Autodesk Fusion 360 part; units mm, degrees
note: some values were not read from the file. Chosen so that the rebuilt part matches the saved one: which bodies a step acts on; that a step has no effect; a side. Set by a fixed rule: which sketch regions a step uses.
(part 2 of 2)
sketch "Schizzo1 (12)" plane through (-2.8, 0, 0) normal (1, 0, 0) x (0, 1, 0) in component "spring"
  line L0 (37.6, 14) -> (48, 14) construction
  line L1 (48, 14) -> (48, 3.6) construction
  line L2 (48, 3.6) -> (37.6, 3.6)
  line L3 (37.6, 3.6) -> (37.6, 14) construction
  line L4 (39.4, 4.4) -> (46.2, 4.4)
  arc A0 (46.2, 4.4) -> (46.2, 6) centre (46.2, 5.2) ccw
  line L5 (46.2, 6) -> (39.4, 6)
  arc A1 (39.4, 6) -> (39.4, 4.4) centre (39.4, 5.2) ccw
  line L6 (39.4, 5.2) -> (46.2, 5.2) construction
  line L7 (46.2, 6.8) -> (39.4, 6.8)
  arc A2 (39.4, 6.8) -> (39.4, 3.6) centre (39.4, 5.2) ccw
  line L8 (39.4, 3.6) -> (46.2, 3.6)
  arc A3 (46.2, 3.6) -> (46.2, 6.8) centre (46.2, 5.2) ccw
  line L9 (42.8, 14) -> (42.8, 3.6) construction
  arc A4 (39.4, 9.2) -> (39.4, 6) centre (39.4, 7.6) ccw
  line L10 (39.4, 6) -> (46.2, 6)
  arc A5 (46.2, 6) -> (46.2, 9.2) centre (46.2, 7.6) ccw
  line L11 (46.2, 9.2) -> (39.4, 9.2)
  arc A6 (46.2, 6.8) -> (46.2, 8.4) centre (46.2, 7.6) ccw
  line L12 (46.2, 8.4) -> (39.4, 8.4)
  arc A7 (39.4, 8.4) -> (39.4, 6.8) centre (39.4, 7.6) ccw
  line L13 (39.4, 6.8) -> (46.2, 6.8)
  arc A8 (39.4, 11.6) -> (39.4, 8.4) centre (39.4, 10) ccw
  line L14 (39.4, 8.4) -> (46.2, 8.4)
  arc A9 (46.2, 8.4) -> (46.2, 11.6) centre (46.2, 10) ccw
  line L15 (46.2, 11.6) -> (39.4, 11.6)
  arc A10 (46.2, 9.2) -> (46.2, 10.8) centre (46.2, 10) ccw
  line L16 (46.2, 10.8) -> (39.4, 10.8)
  arc A11 (39.4, 10.8) -> (39.4, 9.2) centre (39.4, 10) ccw
  line L17 (39.4, 9.2) -> (46.2, 9.2)
  arc A12 (39.4, 14) -> (39.4, 10.8) centre (39.4, 12.4) ccw
  line L18 (39.4, 10.8) -> (46.2, 10.8)
  arc A13 (46.2, 10.8) -> (46.2, 14) centre (46.2, 12.4) ccw
  line L19 (46.2, 14) -> (39.4, 14)
  arc A14 (46.2, 11.6) -> (46.2, 13.2) centre (46.2, 12.4) ccw
  line L20 (46.2, 13.2) -> (39.4, 13.2)
  arc A15 (39.4, 13.2) -> (39.4, 11.6) centre (39.4, 12.4) ccw
  line L21 (39.4, 11.6) -> (46.2, 11.6)
  line L22 (39.4, 12.4) -> (39.4, 5.2)
  line L23 (46.2, 12.4) -> (46.2, 5.2)
  line L24 (39.4, 5.2) -> (39.4, 3.6)
  line L25 (46.2, 12.4) -> (46.2, 14)
  line L26 (37.8, 14) -> (37.8, 3.6)
  line L27 (47.8, 14) -> (47.8, 3.6)
  line L28 (37.8, 14) -> (47.8, 14)
  line L29 (47.8, 14) -> (47.8, 16.2)
  line L30 (47.8, 16.2) -> (37.8, 16.2)
  line L31 (37.8, 16.2) -> (37.8, 14)
  line L32 (37.8, 14) -> (40, 16.2)
  line L33 (37.8, 14) -> (39.4643, 14) construction
  line L34 (47.8, 14) -> (45.6, 16.2)
  line L35 (46.2, 13.2) -> (47.8, 13.2)
  line L36 (39.4, 4.4) -> (37.8, 4.4)
  point P0 (37.6, 14)
  point P1 (48, 3.6)
  dimension "d324" = 1.6
  dimension "d325" = 6.8
  dimension "d326" = 0.8
  dimension "d327" = 1.6
  dimension "d330" = -2.4
  dimension "d331" = 0
  dimension "d332" = 2.2
  dimension "d333" = 45
  constraint horizontal L0
  constraint vertical L1
  constraint horizontal L2
  constraint vertical L3
  constraint coincident P1 L1.end
  constraint coincident P0 L0.start
  constraint tangent L4 A0
  constraint tangent A0 L5
  constraint parallel L4 L5
  constraint tangent L5 A1
  constraint tangent L4 A1
  constraint perpendicular L3 L6
  constraint midpoint L0 L9.start
  constraint midpoint L2 L9.end
  constraint symmetric A1.centre A0.centre L9
  constraint coincident A12.centre A15.centre
  constraint coincident A1.centre L6.start
  constraint coincident A13.centre A14.centre
  constraint coincident A0.centre L6.end
  constraint vertical L26
  constraint tangent A12 L26
  constraint coincident L2 L26.end
  constraint coincident L0 L26.start
  constraint symmetric L9 L26.start L27.start
  constraint symmetric L9 L26.end L27.end
  constraint horizontal L28
  constraint vertical L29
  constraint horizontal L30
  constraint vertical L31
  constraint coincident L26.start L28.start
  constraint coincident L27.start L28.end
  constraint horizontal L33
  constraint coincident L30 L32.end
  constraint symmetric L9 L32.end L34.end
  constraint coincident L27 L35.end
  constraint tangent A14 L35
  constraint coincident L26 L36.end
  constraint tangent A1 L36
  measures "d324" diameter of A0
  measures "d325" distance of A1.centre A0.centre
  measures "d327" distance of L2 A1.centre
  measures "d332" distance of L26.start L30.end
  measures "d333" angle of L32 L33
extrude "Estrusione2''''" add sketch "Schizzo1 (12)" along normal blind 1.6 separate body contours L2 L4 A0 L8 A3 A5 L24 | L2 A2 L26 L36 | A2 L24 L36 | A3 A5 L23 | L5 L7 L10 L13 L22 L23 | A5 A9 L23 | A5 A9 A10 A13 | A2 A4 L22 | A2 A4 A7 A8 | L11 L12 L14 L17 L22 L23 | A9 A13 L23 | A4 A8 L22 | L15 L16 L18 L21 L22 L23 | A13 L25 L35 | A13 L27 L28 L35 | A8 A12 L22 | A8 A12 L19 L20 A15 L25 L28 | L19 L28 L30 L32 L34 | A12 L26 L28 makes body 93 in component "spring"
fillet "Raccordo1''" radius 1 4 edges at (-2, 47.8, 14) (-2, 45.6, 16.2) (-2, 40, 16.2) (-2, 37.8, 14) on bodies 93 in component "spring"
component "drawer" placed x (1, 0, 0) y (0, 1, 0) z (0, 0, 1) at (0, 0, 0)
component "handle" placed x (1, 0, 0) y (0, 1, 0) z (0, 0, 1) at (0, 0, 0)
component "drawer_mount" placed x (1, 0, 0) y (0, 1, 0) z (0, 0, 1) at (0, 0, 0)
component "top_cover" placed x (1, 0, 0) y (0, 1, 0) z (0, 0, 1) at (0, 0, 0)
component "spring" placed x (1, 0, 0) y (0, 1, 0) z (0, 0, 1) at (0, 0, 0)
component "baseplate" placed x (1, 0, 0) y (0, 1, 0) z (0, 0, 1) at (0, 0, 0) in component "drawer"
component "walls" placed x (1, 0, 0) y (0, 1, 0) z (0, 0, 1) at (0, 0, 0) in component "drawer"
component "dividers" placed x (1, 0, 0) y (0, 1, 0) z (0, 0, 1) at (0, 0, 0) in component "drawer"
component " handle recess" placed x (1, 0, 0) y (0, 1, 0) z (0, 0, 1) at (0, 0, 0) in component "drawer"
component "offset" placed x (1, 0, 0) y (0, 1, 0) z (0, 0, 1) at (0, 0, 0) in component "baseplate"
component "foots" placed x (1, 0, 0) y (0, 1, 0) z (0, 0, 1) at (0, 0, 0) in component "drawer_mount"
component "supports" placed x (1, 0, 0) y (0, 1, 0) z (0, 0, 1) at (0, 0, 0) in component "drawer_mount"
component "top_mount_holes" placed x (1, 0, 0) y (0, 1, 0) z (0, 0, 1) at (0, 0, 0) in component "drawer_mount"
component "left" placed x (1, 0, 0) y (0, 1, 0) z (0, 0, 1) at (0, 0, 0) in component "supports"
component "right" placed x (-1, 0, 0) y (0, 1, 0) z (0, 0, -1) at (42, 0, 0) in component "supports"
component "spots" placed x (1, 0, 0) y (0, 1, 0) z (0, 0, 1) at (0, 0, 0) in component "left"
component "spots(Specchio)" placed x (1, 0, 0) y (0, 1, 0) z (0, 0, 1) at (0, 0, 0) in component "right"
component "tracks" placed x (1, 0, 0) y (0, 1, 0) z (0, 0, 1) at (0, 0, 0) in component "top_cover"
equation "baseplate_multiplier = 42 mm"
equation "baseplate_corner_radius = 4 mm"
equation "d3 = baseplate_multiplier"
equation "d4 = baseplate_multiplier"
equation "d5 = baseplate_corner_radius"
equation "d6 = baseplate_corner_radius"
equation "d7 = baseplate_corner_radius"
equation "d8 = baseplate_corner_radius"
equation "d9 = baseplate_multiplier"
equation "d10 = baseplate_multiplier"
equation "drawer_x_unit = 1"
equation "drawer_y_unit = 1"
equation "drawer_z_unit = 1"
equation "drawer_x_unit_computed = max(drawer_x_unit; 1)"
equation "drawer_y_unit_computed = max(drawer_y_unit; 1)"
equation "drawer_z_unit_computed = max(drawer_z_unit; 1)"
equation "d34 = drawer_x_unit_computed + drawer_x_unit_surplus"
equation "d35 = drawer_y_unit_computed + drawer_y_unit_surplus"
equation "d36 = baseplate_multiplier"
equation "d37 = baseplate_multiplier"
equation "drawer_mount_z_multiplier = 21 mm"
equation "drawer_mount_x_multiplier = 70 mm"
equation "drawer_mount_y_multiplier = 56 mm"
equation "drawer_mount_x = drawer_mount_x_multiplier * drawer_x_unit_computed"
equation "drawer_mount_y = drawer_mount_y_multiplier * drawer_y_unit_computed"
equation "drawer_mount_z = drawer_mount_z_multiplier * drawer_z_unit_computed"
equation "drawer_x = drawer_mount_x - 10.4 mm"
equation "drawer_y = drawer_mount_y - 2 mm"
equation "drawer_z = drawer_mount_z - 7 mm"
equation "baseplate_x_offset = drawer_x - ( baseplate_multiplier * drawer_x_unit_computed ) - ( ( 8.8 * 2 ) * 1 mm ) + 0.4 mm"
equation "drawer_x_unit_surplus = ( floor(baseplate_x_offset / 42) ) / mm"
equation "baseplate_y_offset = drawer_y - ( baseplate_multiplier * drawer_y_unit_computed ) - 8 mm"
equation "drawer_y_unit_surplus = ( floor(baseplate_y_offset / 42) ) / mm"
equation "baseplate_x_offset_computed = baseplate_x_offset - ( baseplate_multiplier * drawer_x_unit_surplus )"
equation "baseplate_y_offset_computed = baseplate_y_offset - ( baseplate_multiplier * drawer_y_unit_surplus )"
equation "baseplate_x = baseplate_multiplier * ( drawer_x_unit_computed + drawer_x_unit_surplus )"
equation "baseplate_y = baseplate_multiplier * ( drawer_y_unit_computed + drawer_y_unit_surplus )"
equation "d87 = baseplate_x"
equation "d88 = baseplate_y"
equation "d89 = baseplate_y_offset_computed"
equation "d90 = baseplate_x_offset_computed / 2"
equation "d91 = baseplate_x_offset_computed / 2"
equation "d110 = drawer_z"
equation "d126 = divider_wall_thickness"
equation "d127 = divider_wall_thickness"
equation "divider_wall_thickness = 1.8 mm"
equation "d129 = drawer_z - 4.65 mm"
equation "d131 = drawer_z - 4.65 mm"
equation "d190 = drawer_mount_x"
equation "d191 = drawer_mount_z"
equation "d192 = -drawer_mount_y"
equation "d205 = drawer_mount_z_multiplier / 2"
equation "d208 = drawer_mount_x_multiplier / 2"
equation "d227 = drawer_z_unit_computed"
equation "d229 = -drawer_mount_z_multiplier"
equation "d235 = drawer_x_unit_computed"
equation "d237 = -drawer_mount_x_multiplier"
equation "support_spots_distance = 3 mm"
equation "support_spots_quantity = floor(drawer_mount_y / support_spots_distance)"
equation "d270 = support_spots_quantity"
equation "d272 = drawer_mount_y - 0.4 mm"
equation "d283 = drawer_z_unit_computed"
equation "d285 = drawer_mount_z_multiplier"
equation "d296 = drawer_mount_x_multiplier / 2"
equation "d301 = drawer_x_unit_computed"
equation "d303 = drawer_mount_x_multiplier"
equation "screw_diameter = 3 mm"
equation "screw_length = 16 mm"
equation "d316 = screw_length"
equation "d317 = screw_diameter + 0.5 mm"
equation "d319 = screw_diameter * 2"
equation "d330 = -( 1.6 mm + 0.8 mm )"
named bodies: "vertical_1", "vertical_2", "horizontal", "base", "basic"
